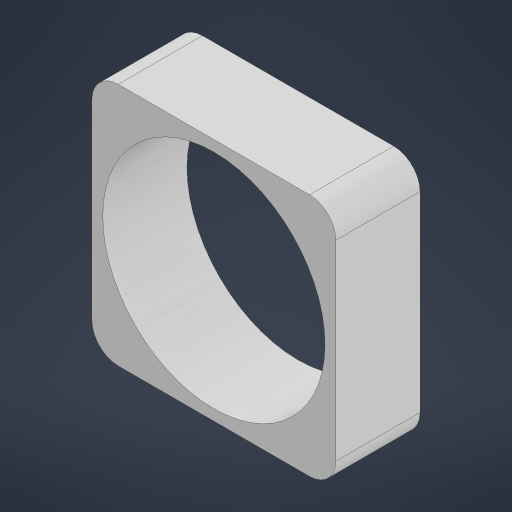
# Autodesk Inventor part: screw_center
Saved by Autodesk Inventor 2024 (Build 280153000, 153)
## iProperties
Created: 2023-11-08
Part Number: screw_center
Material: Generic
Document SubType Name: Modeling
Designer: avere
Density: 1 g/cm^3
Appearance: Default
Author: avere
Autodesk Inventor part; units mm, degrees
ref_plane "YZ Plane" through (0, 0, 0) normal (1, 0, 0) x (0, 1, 0)
ref_plane "XZ Plane" through (0, 0, 0) normal (0, 1, 0) x (-1, 0, 0)
ref_plane "XY Plane" through (0, 0, 0) normal (0, 0, 1) x (1, 0, 0)
sketch "Sketch1" plane through (0, 0, 0) normal (0, 0, 1) x (1, 0, 0)
  line L0 (-5.2597, 91.6776) -> (-5.2597, 95.2844)
  arc A0 (-4.7644, 95.7797) -> (-5.2597, 95.2844) centre (-4.7644, 95.2844) ccw
  line L1 (-4.7644, 95.7797) -> (-1.1576, 95.7797)
  arc A1 (-0.6623, 95.2844) -> (-1.1576, 95.7797) centre (-1.1576, 95.2844) ccw
  line L2 (-0.6623, 95.2844) -> (-0.6623, 91.6776)
  arc A2 (-1.1576, 91.1823) -> (-0.6623, 91.6776) centre (-1.1576, 91.6776) ccw
  line L3 (-1.1576, 91.1823) -> (-4.7644, 91.1823)
  arc A3 (-5.2597, 91.6776) -> (-4.7644, 91.1823) centre (-4.7644, 91.6776) ccw
  circle A4 centre (-2.961, 93.481) radius 2.0955
  point P0 (0, 0)
  dimension "d0" = 4.191
  constraints: 8 end point, 8 point on circle, 5 centre point
  measures "d0" diameter of A4
extrude "Extrusion1" add sketch "Sketch1" along normal blind 1.5875
body "Solid1"
